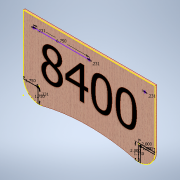
# Autodesk Inventor part: FTC Outside Panels
Saved by Autodesk Inventor 2020 (Build 240168000, 168)
## iProperties
Created: 2022-09-23
Part Number: FTC Outside Panels
Material: Wood (Oak)
Document SubType Name: Modeling
Designer: Jason
Density: 0.76 g/cm^3
Appearance: White Oak - Natural Medium Gloss
Author: Jason
Autodesk Inventor part; units mm, degrees
ref_plane "YZ Plane" through (0, 0, 0) normal (1, 0, 0) x (0, 1, 0)
ref_plane "XZ Plane" through (0, 0, 0) normal (0, 1, 0) x (-1, 0, 0)
ref_plane "XY Plane" through (0, 0, 0) normal (0, 0, 1) x (1, 0, 0)
sketch "Sketch1" plane through (0, 0, 0) normal (0, 0, 1) x (1, 0, 0)
  line L0 (49.2125, 0) -> (54.6328, 0)
  line L1 (357.1875, 0) -> (350.9902, 0)
  arc A0 (0, 49.2125) -> (65.0875, 2.6308) centre (49.2125, 49.2125) ccw
  arc A1 (345.2239, 1.4763) -> (406.4, 49.2125) centre (357.1875, 49.2125) ccw
  arc A2 (203.2, 19.05) -> (54.6328, 0) centre (202.8115, -566.7686) ccw
  arc A3 (350.9902, 0) -> (345.2239, 1.4763) centre (202.8115, -566.7686) ccw
  arc A4 (65.0875, 2.6308) -> (54.6328, 0) centre (202.8115, -566.7686) ccw
  arc A5 (350.9902, 0) -> (203.2, 19.05) centre (202.8115, -566.7686) ccw
  line L2 (0, 49.2125) -> (0, 228.6)
  line L3 (406.4, 228.6) -> (406.4, 49.2125)
  line L4 (0, 228.6) -> (406.4, 228.6)
  point P0 (0, 0)
  point P1 (57.0671, 0.6309)
  constraints: 16 point on circle, 10 end point, 6 centre point, 1 perpendicular, 1 vertical
extrude "Extrusion1" add sketch "Sketch1" along normal blind 5.5563 contours A0 L2 L4 L3 A1 A5 A2
sketch "Sketch4" plane through (0, 0, 5.5563) normal (0, 0, 1) x (1, 0, 0)
  line L0 (406.4, 228.6) -> (0, 228.6) projected
  line L1 (0, 228.6) -> (0, 49.2125) projected
  circle A0 centre (31.75, 196.85) radius 2.9337
  line L2 (406.4, 49.2125) -> (406.4, 228.6) projected
  circle A1 centre (374.65, 196.85) radius 2.9337
  line L3 (31.75, 196.85) -> (203.2, 196.85)
  circle A2 centre (203.2, 196.85) radius 2.9337
  line L4 (51.1152, 176.6695) -> (357.0209, 176.6695) construction
  line L5 (357.0209, 176.6695) -> (357.0209, 65.074) construction
  line L6 (357.0209, 65.074) -> (51.1152, 65.074) construction
  line L7 (51.1152, 65.074) -> (51.1152, 176.6695) construction
  line L8 (355.5735, 0.0265) -> (355.5735, 50.8265)
  line L9 (355.5735, 50.8265) -> (406.3735, 50.8265)
  arc A3 (345.2239, 1.4763) -> (406.4, 49.2125) centre (357.1875, 49.2125) ccw projected
  line L10 (361.7391, 0.2109) -> (361.7391, 44.6609)
  line L11 (361.7391, 44.6609) -> (406.1891, 44.6609)
  circle A4 centre (361.7391, 44.6609) radius 2.9337
  line L12 (0.2109, 44.6609) -> (44.6609, 44.6609)
  line L13 (44.6609, 44.6609) -> (44.6609, 0.2109)
  arc A5 (0, 49.2125) -> (57.0671, 0.6309) centre (49.2125, 49.2125) ccw projected
  circle A6 centre (44.6609, 44.6609) radius 2.9337
  spline S0 degree 2 poles (89.2358, 70.4588) (81.6611, 70.4588) (69.2287, 74.9871) (64.865, 79.1862) knots 0 0 0 1 2 2 2
  spline S1 degree 2 poles (64.865, 79.1862) (60.5836, 83.3029) (56.1376, 94.5003) (56.1376, 100.84) knots 0 0 0 1 2 2 2
  spline S2 degree 2 poles (56.1376, 100.84) (56.1376, 109.0734) (64.9473, 122.9055) (73.3454, 127.0221) knots 0 0 0 1 2 2 2
  line L14 (73.3454, 127.0221) -> (73.3454, 127.4338)
  spline S3 degree 2 poles (73.3454, 127.4338) (65.853, 131.7975) (58.6076, 142.1716) (58.6076, 149.911) knots 0 0 0 1 2 2 2
  spline S4 degree 2 poles (58.6076, 149.911) (58.6076, 161.3554) (75.8977, 176.6695) (89.2358, 176.6695) knots 0 0 0 1 2 2 2
  spline S5 degree 2 poles (89.2358, 176.6695) (103.0679, 176.6695) (119.7817, 162.1787) (119.7817, 150.8166) knots 0 0 0 1 2 2 2
  spline S6 degree 2 poles (119.7817, 150.8166) (119.7817, 143.9829) (111.7953, 130.6448) (104.3029, 126.8575) knots 0 0 0 1 2 2 2
  line L15 (104.3029, 126.8575) -> (104.3029, 126.4458)
  spline S7 degree 2 poles (104.3029, 126.4458) (113.195, 122.3291) (122.334, 110.473) (122.334, 101.087) knots 0 0 0 1 2 2 2
  spline S8 degree 2 poles (122.334, 101.087) (122.334, 88.0782) (103.3972, 70.4588) (89.2358, 70.4588) knots 0 0 0 1 2 2 2
  spline S9 degree 2 poles (108.3373, 99.7696) (108.3373, 106.027) (103.3972, 113.4371) (96.3988, 117.2244) knots 0 0 0 1 2 2 2
  spline S10 degree 2 poles (96.3988, 117.2244) (94.0935, 118.5418) (86.3541, 121.5881) (81.4964, 123.5641) knots 0 0 0 1 2 2 2
  spline S11 degree 2 poles (81.4964, 123.5641) (75.8977, 119.8591) (69.8873, 108.8264) (69.8873, 101.828) knots 0 0 0 1 2 2 2
  spline S12 degree 2 poles (69.8873, 101.828) (69.8873, 92.6066) (81.0024, 80.5858) (89.4005, 80.5858) knots 0 0 0 1 2 2 2
  spline S13 degree 2 poles (89.4005, 80.5858) (97.9632, 80.5858) (108.3373, 90.8776) (108.3373, 99.7696) knots 0 0 0 1 2 2 2
  spline S14 degree 2 poles (106.4436, 150.652) (106.4436, 157.4857) (97.3045, 166.6247) (89.1535, 166.6247) knots 0 0 0 1 2 2 2
  spline S15 degree 2 poles (89.1535, 166.6247) (81.7434, 166.6247) (72.275, 158.4737) (72.275, 151.4753) knots 0 0 0 1 2 2 2
  spline S16 degree 2 poles (72.275, 151.4753) (72.275, 146.4529) (77.1327, 139.4546) (81.9904, 136.6552) knots 0 0 0 1 2 2 2
  spline S17 degree 2 poles (81.9904, 136.6552) (84.0488, 135.5025) (92.7762, 131.4682) (96.3165, 130.3155) knots 0 0 0 1 2 2 2
  spline S18 degree 2 poles (96.3165, 130.3155) (102.2445, 134.8439) (106.4436, 144.4769) (106.4436, 150.652) knots 0 0 0 1 2 2 2
  line L16 (200.1395, 107.6737) -> (188.0364, 107.6737)
  line L17 (188.0364, 107.6737) -> (188.0364, 72.7641)
  line L18 (188.0364, 72.7641) -> (174.9454, 72.7641)
  line L19 (174.9454, 72.7641) -> (174.9454, 107.6737)
  line L20 (174.9454, 107.6737) -> (130.0734, 107.6737)
  line L21 (130.0734, 107.6737) -> (130.0734, 121.9998)
  line L22 (130.0734, 121.9998) -> (175.5217, 174.3641)
  line L23 (175.5217, 174.3641) -> (188.0364, 174.3641)
  line L24 (188.0364, 174.3641) -> (188.0364, 118.6241)
  line L25 (188.0364, 118.6241) -> (200.1395, 118.6241)
  line L26 (200.1395, 118.6241) -> (200.1395, 107.6737)
  line L27 (174.9454, 118.6241) -> (174.9454, 158.309)
  line L28 (174.9454, 158.309) -> (140.7768, 118.6241)
  line L29 (140.7768, 118.6241) -> (174.9454, 118.6241)
  spline S19 degree 2 poles (274.24, 123.5641) (274.24, 96.2293) (258.3496, 70.6234) (241.8005, 70.6234) knots 0 0 0 1 2 2 2
  spline S20 degree 2 poles (241.8005, 70.6234) (225.0043, 70.6234) (209.2786, 96.7233) (209.2786, 123.4818) knots 0 0 0 1 2 2 2
  spline S21 degree 2 poles (209.2786, 123.4818) (209.2786, 150.9813) (225.169, 176.4225) (241.8005, 176.4225) knots 0 0 0 1 2 2 2
  spline S22 degree 2 poles (241.8005, 176.4225) (258.5142, 176.4225) (274.24, 150.0756) (274.24, 123.5641) knots 0 0 0 1 2 2 2
  spline S23 degree 2 poles (256.7852, 92.6066) (258.7612, 97.629) (260.4079, 113.1077) (260.4079, 123.5641) knots 0 0 0 1 2 2 2
  spline S24 degree 2 poles (260.4079, 123.5641) (260.4079, 134.0205) (258.7612, 149.417) (256.7029, 154.604) knots 0 0 0 1 2 2 2
  spline S25 degree 2 poles (256.7029, 154.604) (254.6445, 159.791) (247.4815, 165.1427) (241.8005, 165.1427) knots 0 0 0 1 2 2 2
  spline S26 degree 2 poles (241.8005, 165.1427) (236.1194, 165.1427) (228.7917, 159.791) (226.651, 154.4393) knots 0 0 0 1 2 2 2
  spline S27 degree 2 poles (226.651, 154.4393) (224.5927, 149.2523) (223.1107, 133.4442) (223.1107, 123.4818) knots 0 0 0 1 2 2 2
  spline S28 degree 2 poles (223.1107, 123.4818) (223.1107, 112.7784) (224.428, 98.4523) (226.5687, 92.8536) knots 0 0 0 1 2 2 2
  spline S29 degree 2 poles (226.5687, 92.8536) (228.5447, 87.5842) (235.8724, 81.9032) (241.8005, 81.9032) knots 0 0 0 1 2 2 2
  spline S30 degree 2 poles (241.8005, 81.9032) (247.3992, 81.9032) (254.7269, 87.2549) (256.7852, 92.6066) knots 0 0 0 1 2 2 2
  spline S31 degree 2 poles (350.4812, 123.5641) (350.4812, 96.2293) (334.5907, 70.6234) (318.0416, 70.6234) knots 0 0 0 1 2 2 2
  spline S32 degree 2 poles (318.0416, 70.6234) (301.2455, 70.6234) (285.5197, 96.7233) (285.5197, 123.4818) knots 0 0 0 1 2 2 2
  spline S33 degree 2 poles (285.5197, 123.4818) (285.5197, 150.9813) (301.4102, 176.4225) (318.0416, 176.4225) knots 0 0 0 1 2 2 2
  spline S34 degree 2 poles (318.0416, 176.4225) (334.7554, 176.4225) (350.4812, 150.0756) (350.4812, 123.5641) knots 0 0 0 1 2 2 2
  spline S35 degree 2 poles (333.0264, 92.6066) (335.0024, 97.629) (336.6491, 113.1077) (336.6491, 123.5641) knots 0 0 0 1 2 2 2
  spline S36 degree 2 poles (336.6491, 123.5641) (336.6491, 134.0205) (335.0024, 149.417) (332.9441, 154.604) knots 0 0 0 1 2 2 2
  spline S37 degree 2 poles (332.9441, 154.604) (330.8857, 159.791) (323.7227, 165.1427) (318.0416, 165.1427) knots 0 0 0 1 2 2 2
  spline S38 degree 2 poles (318.0416, 165.1427) (312.3606, 165.1427) (305.0329, 159.791) (302.8922, 154.4393) knots 0 0 0 1 2 2 2
  spline S39 degree 2 poles (302.8922, 154.4393) (300.8338, 149.2523) (299.3518, 133.4442) (299.3518, 123.4818) knots 0 0 0 1 2 2 2
  spline S40 degree 2 poles (299.3518, 123.4818) (299.3518, 112.7784) (300.6692, 98.4523) (302.8099, 92.8536) knots 0 0 0 1 2 2 2
  spline S41 degree 2 poles (302.8099, 92.8536) (304.7859, 87.5842) (312.1136, 81.9032) (318.0416, 81.9032) knots 0 0 0 1 2 2 2
  spline S42 degree 2 poles (318.0416, 81.9032) (323.6403, 81.9032) (330.968, 87.2549) (333.0264, 92.6066) knots 0 0 0 1 2 2 2
  point P0 (0, 0)
  dimension "d29" = 5.8674
  dimension "d31" = 5.8674
  dimension "d32" = 171.45
  dimension "d33" = 5.8674
  dimension "d47" = 50.8
  dimension "d48" = 50.8
  dimension "d49" = 44.45
  dimension "d50" = 44.45
  dimension "d51" = 5.8674
  dimension "d52" = 44.45
  dimension "d53" = 44.45
  dimension "d54" = 5.8674
  constraints: 14 end point, 6 point on circle, 5 centre point, 3 coincident, 3 perpendicular, 2 horizontal, 2 vertical, 2 other
  measures "d29" diameter of A0
  measures "d31" diameter of A1
  measures "d32" distance of L3.start L3.end
  measures "d33" diameter of A2
  measures "d47" distance of L8.start L8.end
  measures "d48" distance of L8.end L9.end
  measures "d49" distance of L10.start L10.end
  measures "d50" distance of L10.end L11.end
  measures "d51" diameter of A4
  measures "d52" distance of L12.start L12.end
  measures "d53" distance of L12.end L13.end
  measures "d54" diameter of A6
extrude "Extrusion4" cut sketch "Sketch4" against normal blind 5.5626 contours A0 | A1 | A2 | A4 L11 L10 | L10 L11 A4 | A6 L13 L12 | L12 L13 A6
extrude "Extrusion5" cut sketch "Sketch4" against normal blind 2.54 contours S0 S1 S2 L14 S3 S4 S5 S6 L15 S7 S8 | L16 L17 L18 L19 L20 L21 L22 L23 L24 L25 L26 | S19 S20 S21 S22 | S31 S32 S33 S34
body "Solid1"
